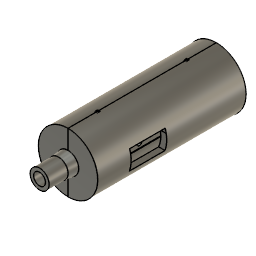
Thermometer top partf3d (Autodesk Fusion 360 design; units mm, degrees)
part number: 2026-05-12-22-40-57-730
Autodesk Fusion 360 part; units mm, degrees
sketch "Sketch15" plane through (0, 0, 0) normal (0, 0, 1) x (1, 0, 0)
sketch "Sketch16" plane through (0, 0, 0) normal (0, 1, 0) x (1, 0, 0)
  circle A0 centre (0, 0) radius 20.0625
  dimension "d43" = 40.125
  constraint coincident A0.centre origin
  measures "d43" diameter of A0
extrude "Extrude8" add sketch "Sketch16" along normal blind 115.2 makes body 1
shell "Shell3" thickness 5 outward yes removed faces 0 bodies 1
split "Split2" by plane through (0, 0, 0) normal (1, 0, 0) bodies 1 makes body 2 at (20.4153, 78.4667, 14.5377)
sketch "Sketch17" plane through (0, 0, 0) normal (-1, 0, 0) x (0, -1, 0)
  line L0 (-115.2, 20.0625) -> (0, 20.0625)
  line L1 (0, 20.0625) -> (0, -20.0625)
  line L2 (0, -20.0625) -> (-115.2, -20.0625)
  line L3 (-115.2, -20.0625) -> (-115.2, 20.0625)
  line L4 (5, 25.0625) -> (-120.2, 25.0625)
  line L5 (-120.2, 25.0625) -> (-120.2, -25.0625)
  line L6 (-120.2, -25.0625) -> (5, -25.0625)
  line L7 (5, -25.0625) -> (5, 25.0625)
  circle A0 centre (-95.2, 22.5625) radius 2.5
  circle A1 centre (-20, 22.5625) radius 2.5
  circle A2 centre (-95.2, -22.5625) radius 2.5
  circle A3 centre (-20, -22.5625) radius 2.5
  dimension "d47" = 5
  dimension "d48" = 2.5
  dimension "d49" = 25
  dimension "d50" = 5
  dimension "d51" = 2.5
  dimension "d52" = 25
  dimension "d53" = 5
  dimension "d54" = 2.5
  dimension "d55" = 5
  measures "d47" diameter of A0
  measures "d48" distance of L4 A0.centre
  measures "d49" distance of L5 A0.centre
  measures "d50" diameter of A1
  measures "d51" distance of L0 A1.centre
  measures "d52" distance of L7 A1.centre
  measures "d53" diameter of A2
  measures "d54" distance of L6 A2.centre
  measures "d55" diameter of A3
extrude "Extrude9" cut sketch "Sketch17" against normal blind 1 contours A0 | A1 | A2 | A3 bodies 2
sketch "Sketch18" plane through (0, 0, 0) normal (1, 0, 0) x (0, 1, 0)
sketch "Sketch19" plane through (0, 0, 0) normal (1, 0, 0) x (0, 1, 0)
  circle A0 centre (20, 22.5625) radius 2.5
  line L0 (120.2, 25.0625) -> (-5, 25.0625)
  line L1 (-5, 25.0625) -> (-5, -25.0625)
  circle A1 centre (95.2, 22.5625) radius 2.5
  line L2 (0, 20.0625) -> (115.2, 20.0625)
  line L3 (120.2, -25.0625) -> (120.2, 25.0625)
  circle A2 centre (20, -22.5625) radius 2.5
  line L4 (115.2, -20.0625) -> (0, -20.0625)
  circle A3 centre (95.2, -22.5625) radius 2.5
  dimension "d58" = 5
  dimension "d59" = 2.5
  dimension "d60" = 25
  dimension "d61" = 5
  dimension "d62" = 2.5
  dimension "d63" = 25
  dimension "d64" = 5
  dimension "d65" = 2.5
  dimension "d66" = 25
  dimension "d67" = 5
  measures "d58" diameter of A0
  measures "d59" distance of A0.centre L0
  measures "d60" distance of A0.centre L1
  measures "d61" diameter of A1
  measures "d62" distance of A1.centre L2
  measures "d63" distance of A1.centre L3
  measures "d64" diameter of A2
  measures "d65" distance of A2.centre L4
  measures "d66" distance of L1 A2.centre
  measures "d67" diameter of A3
extrude "Extrude10" cut sketch "Sketch19" against normal blind 1.1 contours A0 | A1 | A2 | A3 bodies 1
sketch "Sketch20" plane through (0, 0, 0) normal (1, 0, 0) x (0, 1, 0)
  line L0 (115.2, -19.5) -> (0, -19.5)
  line L1 (0, -19.5) -> (0, 19)
  line L2 (0, 19) -> (115.2, 19)
  line L3 (115.2, 19) -> (115.2, -19.5)
  constraint horizontal L0
  constraint vertical L1
  constraint horizontal L2
  constraint vertical L3
extrude "Extrude11" add sketch "Sketch20" against normal blind 5 separate body makes body 3
sketch "Sketch21" plane through (0, 0, 0) normal (1, 0, 0) x (0, 1, 0)
  line L0 (115.2, 19) -> (0, 19)
  line L1 (0, 19) -> (0, -19.5)
  line L2 (0, -19.5) -> (115.2, -19.5)
  line L3 (115.2, -19.5) -> (115.2, 19)
  line L4 (110, -13.5) -> (3.6171, -13.5)
  line L5 (3.6171, -13.5) -> (3.6171, 13)
  line L6 (3.6171, 13) -> (110, 13)
  line L7 (110, 13) -> (110, -13.5)
  dimension "d72" = 26.5
  dimension "d73" = 6
  constraint horizontal L4
  constraint vertical L5
  constraint horizontal L6
  constraint vertical L7
  measures "d72" distance of L4.start L6.end
  measures "d73" distance of L2 L4
extrude "Extrude12" cut sketch "Sketch21" against normal blind 4 contours L4 L5 L6 L7 bodies 3
sketch "Sketch22" plane through (0, 0, 0) normal (1, 0, 0) x (0, 1, 0)
  line L0 (3.6171, -13.5) -> (3.6171, 13)
  line L1 (3.6171, 13) -> (110, 13)
  line L2 (110, 13) -> (110, -13.5)
  line L3 (110, -13.5) -> (3.6171, -13.5)
  line L4 (115.2, 19) -> (0, 19)
  line L5 (0, 19) -> (0, -19.5)
  line L6 (0, -19.5) -> (115.2, -19.5)
  line L7 (115.2, -19.5) -> (115.2, 19)
  line L8 (0, -13.5509) -> (115.2, -13.5509)
  line L9 (115.2, -13.5509) -> (115.2, 13)
  line L10 (115.2, 13) -> (0, 13)
  line L11 (0, 13) -> (0, -13.5509)
  constraint horizontal L8
  constraint vertical L9
  constraint horizontal L10
  constraint vertical L11
  constraint coincident L7 L9.end
  constraint coincident L5 L8.start
extrude "Extrude13" cut sketch "Sketch22" against normal blind 4 contours L0 L2 L3 L5 L7 L8 L9 L10 L11 bodies 3
sketch "Sketch23" plane through (0, 0, 0) normal (1, 0, 0) x (0, 1, 0)
  line L0 (115.2, -13.5509) -> (0, -13.5509)
  line L1 (0, -13.5509) -> (0, -19.5)
  line L2 (0, -19.5) -> (115.2, -19.5)
  line L3 (115.2, -19.5) -> (115.2, -13.5509)
  circle A0 centre (55.2, -15.7509) radius 2
  circle A1 centre (55.2, 15.2491) radius 2
  dimension "d78" = 4
  dimension "d79" = 60
  dimension "d80" = 4
  dimension "d81" = 31
  dimension "d82" = 2.2
  measures "d78" diameter of A0
  measures "d79" distance of L3 A0.centre
  measures "d80" diameter of A1
  measures "d81" distance of A0.centre A1.centre
  measures "d82" distance of L0 A0.centre
extrude "Extrude14" cut sketch "Sketch23" against normal blind 5 contours A0 | A1 bodies 3
sketch "Sketch24" plane through (0, 0, 0) normal (1, 0, 0) x (0, 1, 0)
  line L0 (23.2, -8.4625) -> (53.2, -8.4625)
  line L1 (53.2, -8.4625) -> (53.2, 4.5375)
  line L2 (53.2, 4.5375) -> (23.2, 4.5375)
  line L3 (23.2, 4.5375) -> (23.2, -8.4625)
  line L4 (95.2, -20.0625) -> (20, -20.0625)
  line L5 (0, -19.5) -> (0, 19)
  dimension "d85" = 30
  dimension "d86" = 13
  dimension "d87" = 11.6
  dimension "d88" = 53.2
  constraint horizontal L0
  constraint vertical L1
  constraint horizontal L2
  constraint vertical L3
  measures "d85" distance of L0.start L0.end
  measures "d86" distance of L0.start L2.end
  measures "d87" distance of L0 L4
  measures "d88" distance of L1 L5
extrude "Extrude15" cut sketch "Sketch24" along normal mid plane 60 bodies 2 3
sketch "Sketch25" plane through (0, -5, 0) normal (0, -1, 0) x (1, 0, 0)
  line L0 (0, 25.0625) -> (0, -25.0625)
  arc A0 (0, -25.0625) -> (0, 25.0625) centre (0, 0) ccw
  circle A1 centre (0, 0) radius 3.1
  dimension "d91" = 6.2
  constraint coincident A0.centre A1.centre
  measures "d91" diameter of A1
extrude "Extrude16" cut sketch "Sketch25" against normal blind 5 contours L0 A1 | L0 A1 bodies 1 2
sketch "Sketch26" plane through (0, -5, 0) normal (0, -1, 0) x (1, 0, 0)
  arc A0 (0, 3.1) -> (0, -3.1) centre (0, 0) ccw
  line L0 (0, 3.1) -> (0, 25.0625)
  arc A1 (0, 25.0625) -> (0, -25.0625) centre (0, 0) ccw
  line L1 (0, -25.0625) -> (0, -3.1)
  circle A2 centre (0, 0) radius 9
  circle A3 centre (0, 0) radius 4.335
  dimension "d94" = 18
  dimension "d104" = 8.67
  constraint coincident A0.centre A1.centre
  constraint concentric A2 A3
  measures "d94" diameter of A2
  measures "d104" diameter of A3
extrude "Extrude17" add sketch "Sketch26" along normal blind 8 draft -6.7 separate body contours A0 L0 L1 A3 | A0 L0 L1 A3 | L0 L1 A2 A3 | L0 L1 A2 A3 makes body 4
sketch "Sketch27" plane through (0, -13, 0) normal (0, -1, 0) x (1, 0, 0)
  circle A0 centre (0, 0) radius 8.0602
  circle A1 centre (0, 0) radius 3.1
  dimension "d97" = 6.2
  constraint coincident A0.centre A1.centre
  measures "d97" diameter of A1
extrude "Extrude18" cut sketch "Sketch27" against normal blind 8 contours A1 bodies 4
sketch "Sketch28" plane through (0, 0, 0) normal (1, 0, 0) x (0, 1, 0)
  line L0 (-5, 3.1) -> (0, 3.1)
  line L1 (0, 3.1) -> (0, 20.0625)
  line L2 (0, 20.0625) -> (20, 20.0625)
  arc A0 (20, 25.0625) -> (20, 20.0625) centre (20, 22.5625) ccw
  line L3 (20, 25.0625) -> (-5, 25.0625)
  line L4 (-5, 25.0625) -> (-5, 3.1)
  line L5 (-3.0274, 20.0625) -> (0, 20.0625)
  line L6 (0, 20.0625) -> (0, -20)
  line L7 (0, -20) -> (-3.0274, -20)
  line L8 (-3.0274, -20) -> (-3.0274, 20.0625)
  constraint horizontal L5
  constraint vertical L6
  constraint horizontal L7
  constraint vertical L8
extrude "Extrude19" cut sketch "Sketch28" against normal blind 2 contours L0 L1 L5 L6 L8 | L0 L6 L7 L8 bodies 1
sketch "Sketch29" plane through (-4, 0, 0) normal (1, 0, 0) x (0, 1, 0)
  line L0 (23.2, 4.5375) -> (53.2, 4.5375)
  line L1 (53.2, 4.5375) -> (53.2, -8.4625)
  line L2 (53.2, -8.4625) -> (23.2, -8.4625)
  line L3 (23.2, -8.4625) -> (23.2, 4.5375)
  line L4 (115.2, 13) -> (0, 13)
  line L5 (0, 13) -> (0, -13.5509)
  line L6 (0, -13.5509) -> (115.2, -13.5509)
  line L7 (115.2, -13.5509) -> (115.2, 13)
  line L8 (23.2, 4.5375) -> (53.1903, 4.5375)
  line L9 (53.1903, 4.5375) -> (53.1903, 7.9553)
  line L10 (53.1903, 7.9553) -> (23.2, 7.9553)
  line L11 (23.2, 7.9553) -> (23.2, 4.5375)
  constraint horizontal L8
  constraint vertical L9
  constraint horizontal L10
  constraint vertical L11
  constraint coincident L0.start L3.end
extrude "Extrude20" cut sketch "Sketch29" along normal blind 35 contours L0 L8 L9 L10 L11 bodies 2
split "Split3" by plane through (0, 0, 0) normal (1, 0, 0) bodies 4 makes body 5 at (6.9923, -5, -0.574)
hole "Hole2" at (0, -13, 0) direction (0, 1, 0) diameter 10 depth 11 tip angle 118 bodies 1 4 5
delete_face "DeleteFace1" 1 faces at (-3.9605, -1.6195, 1.8391) on bodies 1
hole "Hole3" at (0, -5, 0) direction (0, 1, 0) diameter 10 depth 5 tip angle 180 bodies 2
extrude "Extrude21" add 2 faces at (-0.4004, -13, 7.0101) (2.4489, -13, -6.5807) along direction (0, -1, 0) blind 16 on bodies 4 5 bodies 4 5
sketch "Sketch2" plane through (0, 0, 0) normal (0, 1, 0) x (1, 0, 0)
  line L0 (20.5, -2) -> (-20.5, -2)
  line L1 (-20.5, -2) -> (-20.5, -118)
  line L2 (-20.5, -118) -> (20.5, -118)
  line L3 (20.5, -118) -> (20.5, -2)
  line L4 (-22.5, -120) -> (-22.5, 0)
  line L5 (-22.5, 0) -> (22.5, 0)
  line L6 (22.5, 0) -> (22.5, -120)
  line L7 (22.5, -120) -> (-22.5, -120)
  line L8 (21.5, -1) -> (21.5, -119)
  line L9 (21.5, -119) -> (-21.5, -119)
  line L10 (-21.5, -119) -> (-21.5, -1)
  line L11 (-21.5, -1) -> (21.5, -1)
  dimension "d9" = 1
sketch "Sketch3" plane through (0, 0, 0) normal (0, 1, 0) x (1, 0, 0)
sketch "Sketch4" plane through (0, 0, 0) normal (0, 0, 1) x (1, 0, 0)
  circle A0 centre (0, 0.7) radius 2.85
  dimension "d10" = 5.7
  measures "d10" diameter of A0
sketch "Sketch5" plane through (0, 0, 0) normal (0, 0, 1) x (1, 0, 0)
  circle A0 centre (0, 0.75) radius 2.85
  dimension "d13" = 5.7
  measures "d13" diameter of A0
sketch "Sketch6" plane through (0, 0, 0) normal (0, 1, 0) x (1, 0, 0)
ref_plane "WorkPlane1" through (0, -22.5, 21.1578) normal (0, -1, 0) x (-1, 0, 0)
sketch "Sketch7" plane through (0, -22.5, 0) normal (0, -1, 0) x (-1, 0, 0)
  line L0 (5.75, -52.4) -> (-5.75, -52.4)
  line L1 (-5.75, -52.4) -> (-5.75, -30.02)
  line L2 (-5.75, -30.02) -> (5.75, -30.02)
  line L3 (5.75, -30.02) -> (5.75, -52.4)
  line L4 (-20.5, -118) -> (-20.5, -2)
  line L5 (-20.5, -2) -> (20.5, -2)
  dimension "d20" = 11.5
  dimension "d21" = 22.38
  dimension "d22" = 14.75
  dimension "d23" = 28.02
  constraint horizontal L0
  constraint vertical L1
  constraint horizontal L2
  constraint vertical L3
  measures "d20" distance of L0.start L0.end
  measures "d21" distance of L0.start L2.end
  measures "d22" distance of L1 L4
  measures "d23" distance of L2 L5
sketch "Sketch8" plane through (0, 0, 0) normal (0, 1, 0) x (1, 0, 0)
  line L0 (-6.8848, -54.404) -> (6.899, -54.404)
  line L1 (6.899, -54.404) -> (6.899, -23.7134)
  line L2 (6.899, -23.7134) -> (-6.8848, -23.7134)
  line L3 (-6.8848, -23.7134) -> (-6.8848, -54.404)
  constraint horizontal L0
  constraint vertical L1
  constraint horizontal L2
  constraint vertical L3
sketch "Sketch9" plane through (0, 0, 0) normal (0, 1, 0) x (1, 0, 0)
sketch "Sketch10" plane through (0, 0, 120) normal (0, 0, 1) x (-1, 0, 0)
  line L0 (-22.5, 0) -> (22.5, 0)
  arc A0 (22.5, 0) -> (-22.5, 0) centre (0, 0) ccw
sketch "Sketch11" plane through (0, 0, 0) normal (1, 0, 0) x (0, 1, 0)
  line L0 (-10, 120) -> (-10, 127.2371)
  line L1 (-10, 127.2371) -> (27.6494, 127.2371)
  line L2 (27.6494, 127.2371) -> (27.6494, 112)
  constraint vertical L0
  constraint perpendicular L0 L1
  constraint perpendicular L1 L2
sketch "Sketch12" plane through (0, 0, 120) normal (0, 0, 1) x (-1, 0, 0)
  line L0 (-2, 11) -> (2, 11)
  line L1 (2, 11) -> (2, 9)
  line L2 (2, 9) -> (-2, 9)
  line L3 (-2, 9) -> (-2, 11)
  constraint horizontal L0
  constraint vertical L1
  constraint horizontal L2
  constraint vertical L3
sketch "Sketch13" plane through (0, 28.6494, 0) normal (0, 1, 0) x (-1, 0, 0)
  line L0 (-1, 127.2371) -> (-1, 113)
  line L1 (-1, 113) -> (1, 113)
  line L2 (1, 113) -> (1, 127.2371)
  line L3 (1, 127.2371) -> (-1, 127.2371)
  circle A0 centre (0, 115) radius 1
  dimension "d36" = 2
  measures "d36" diameter of A0
sketch "Sketch14" plane through (0, 28.6494, 0) normal (0, 1, 0) x (-1, 0, 0)
